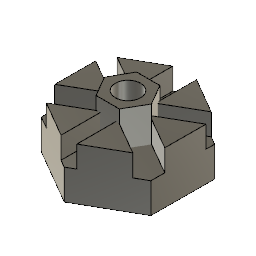
PulseCouplingCapacitorJig (Autodesk Fusion 360 design; units mm, degrees)
Autodesk Fusion 360 part; units mm, degrees
sketch "Sketch1" plane through (0, 0, 0) normal (0, 0, 1) x (1, 0, 0)
  line L0 (-6.3336, 3.6944) -> (-6.3663, -3.6379)
  line L1 (-6.3663, -3.6379) -> (-0.0326, -7.3323)
  line L2 (-0.0326, -7.3323) -> (6.3336, -3.6944)
  line L3 (6.3336, -3.6944) -> (6.3663, 3.6379)
  line L4 (6.3663, 3.6379) -> (0.0326, 7.3323)
  line L5 (0.0326, 7.3323) -> (-6.3336, 3.6944)
  line L6 (-1.35, 2.3383) -> (1.35, 2.3383)
  line L7 (1.35, 2.3383) -> (2.7, 0)
  line L8 (2.7, 0) -> (1.35, -2.3383)
  line L9 (1.35, -2.3383) -> (-1.35, -2.3383)
  line L10 (-1.35, -2.3383) -> (-2.7, 0)
  line L11 (-2.7, 0) -> (-1.35, 2.3383)
  line L12 (-2.025, 1.1691) -> (0, 0)
  point P0 (0, 2.3383)
  point P1 (-2.025, 1.1691)
  dimension "d3" = 12.7
  dimension "d34" = 2.7
  dimension "d35" = 2.7
  dimension "d36" = 120
  dimension "d37" = 120
  constraint horizontal L6
  constraint parallel L6 L9
  constraint equal L7 L11
  constraint equal L9 L11
  constraint equal L6 L10
  constraint equal L8 L10
  constraint midpoint L6 P0
  constraint midpoint L11 P1
  constraint coincident P1 L12.start
  constraint coincident L12.end origin
  constraint perpendicular L11 L12
  constraint vertical L12.end P0
  measures "d3" distance of L2 L5
  measures "d34" distance of L6.end L7.end
  measures "d35" distance of L7.end L8.end
  measures "d36" angle of L7 L8
  measures "d37" angle of L6 L7
extrude "Extrude1" add sketch "Sketch1" along normal blind 6 contours L0 L1 L2 L3 L4 L5 | L6 L7 L8 L9 L10 L11 makes body 1
sketch "Sketch2" plane through (0, 0, 6) normal (0, 0, 1) x (-1, 0, 0)
  line L0 (-0.0326, -7.3323) -> (6.3336, -3.6944)
  line L1 (6.3336, -3.6944) -> (6.3663, 3.6379)
  line L2 (6.3663, 3.6379) -> (0.0326, 7.3323)
  line L3 (0.0326, 7.3323) -> (-6.3336, 3.6944)
  line L4 (-6.3336, 3.6944) -> (-6.3663, -3.6379)
  line L5 (-6.3663, -3.6379) -> (-0.0326, -7.3323)
  line L6 (1.35, -7.3323) -> (-1.35, -7.3323)
  line L7 (-1.35, -7.3323) -> (-1.35, 0)
  line L8 (-1.35, 0) -> (1.35, 0)
  line L9 (1.35, 0) -> (1.35, -7.3323)
  line L10 (0, -1.75) -> (0, -22.5)
  line L11 (0.9, 0) -> (-0.9, 0)
  line L12 (-0.9, 0) -> (-0.9, 7.3323)
  line L13 (-0.9, 7.3323) -> (0.9, 7.3323)
  line L14 (0.9, 7.3323) -> (0.9, 0)
  dimension "d6" = 2.7
  dimension "d29" = 1.8
  constraint horizontal L6
  constraint vertical L7
  constraint horizontal L8
  constraint vertical L9
  constraint coincident L0.start L6
  constraint coincident origin L8
  constraint symmetric L7 L9 L10
  constraint horizontal L11
  constraint vertical L12
  constraint horizontal L13
  constraint vertical L14
  constraint coincident L8 L11.start
  constraint symmetric L10 L12 L14
  constraint coincident L2.end L13
  measures "d6" distance of L7.end L8.end
  measures "d29" distance of L12.end L13.end
extrude "Extrude2" cut sketch "Sketch2" against normal blind 2.5 contours L0 L5 L7 L8 L9 L11 bodies 1
extrude "Extrude3" add sketch "Sketch1" along normal blind 10 separate body contours L6 L7 L8 L9 L10 L11 makes body 2
hole "Hole1" at (0, 0, 0) direction (0, 0, 1) diameter 2.9 end through all bodies 2 1
extrude "Extrude4" add sketch "Sketch1" along normal blind 7.5 separate body contours L6 L7 L8 L9 L10 L11 makes body 3
sketch "Sketch3" plane through (0, 0, 0) normal (0, 0, -1) x (1, 0, 0)
  line L0 (-1.35, 2.3383) -> (-2.7, 0)
  line L1 (-2.7, 0) -> (-1.35, -2.3383)
  line L2 (-1.35, -2.3383) -> (1.35, -2.3383)
  line L3 (1.35, -2.3383) -> (2.7, 0)
  line L4 (2.7, 0) -> (1.35, 2.3383)
  line L5 (1.35, 2.3383) -> (-1.35, 2.3383)
hole "Hole2" at (0, 0, 0) direction (0, 0, 1) diameter 2.9 end through all bodies 3
sketch "Sketch4" plane through (0, 0, 0) normal (0, 0, -1) x (1, 0, 0)
  circle A0 centre (0, 0) radius 1.45
  line L0 (-6.3336, -3.6944) -> (0.0326, -7.3323)
  line L1 (0.0326, -7.3323) -> (6.3663, -3.6379)
  line L2 (6.3663, -3.6379) -> (6.3336, 3.6944)
  line L3 (6.3336, 3.6944) -> (-0.0326, 7.3323)
  line L4 (-0.0326, 7.3323) -> (-6.3663, 3.6379)
  line L5 (-6.3663, 3.6379) -> (-6.3336, -3.6944)
  line L6 (-1.4434, 2.5) -> (-2.8868, 0)
  line L7 (-2.8868, 0) -> (-1.4434, -2.5)
  line L8 (-1.4434, -2.5) -> (1.4434, -2.5)
  line L9 (1.4434, -2.5) -> (2.8868, 0)
  line L10 (2.8868, 0) -> (1.4434, 2.5)
  line L11 (1.4434, 2.5) -> (-1.4434, 2.5)
  dimension "d26" = 5
  constraint coincident A0.centre origin
  measures "d26" distance of L8 L11
extrude "Extrude5" cut sketch "Sketch4" against normal blind 2 contours A0 | L6 L7 L8 L9 L10 L11 bodies 1 3
pattern_circular "C-Pattern1" count 3 over 360 about axis through (0, 0, 1.75) along (0, 0, 1) of "Extrude2"
extrude "Extrude6" cut sketch "Sketch2" against normal up to surface (2.5 mm away) contours L2 L3 L8 L11 L12 L14 bodies 1
pattern_circular "C-Pattern2" count 3 over 360 about axis through (0, 0, 1.75) along (0, 0, 1) of "Extrude6"
hidden bodies 2
